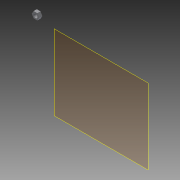
# Autodesk Inventor part: m5_nut
Saved by Autodesk Inventor 2014 (Build 180170000, 170)
## iProperties
Created: 2014-02-14
Part Number: m5_nut
Material: Generic
Document SubType Name: Modeling
Designer: stephen
Density: 1 g/cm^3
Appearance: Default
Author: stephen
Autodesk Inventor part; units mm, degrees
ref_plane "YZ Plane" through (0, 0, 0) normal (1, 0, 0) x (0, 1, 0)
ref_plane "XZ Plane" through (0, 0, 0) normal (0, 1, 0) x (-1, 0, 0)
ref_plane "XY Plane" through (0, 0, 0) normal (0, 0, 1) x (1, 0, 0)
ref_plane "Work Plane2" through (-37.9568, -6.3739, 16.6205) normal (0.2239, -0.0206, 0.9744) x (0.9746, 0.0023, -0.2239)
sketch "Sketch1" plane through (-37.9568, -6.3739, 16.6205) normal (0.2239, -0.0206, 0.9744) x (0.9746, 0.0023, -0.2239)
  circle A0 centre (40.7292, 6.1193) radius 2.5
  line L0 (45.348, 6.1193) -> (43.0386, 2.1193)
  line L1 (43.0386, 2.1193) -> (38.4198, 2.1193)
  line L2 (38.4198, 2.1193) -> (36.1104, 6.1193)
  line L3 (36.1104, 6.1193) -> (38.4198, 10.1193)
  line L4 (38.4198, 10.1193) -> (43.0386, 10.1193)
  line L5 (43.0386, 10.1193) -> (45.348, 6.1193)
  point P0 (40.7292, 6.1193)
  dimension "d0" = 5
  dimension "d1" = 8
  constraints: 12 end point, 2 coincident, 1 centre point, 13 other
  measures "d0" diameter of A0
  measures "d1" distance between parallel lines of L1 L4
extrude "Extrusion1" add sketch "Sketch1" along normal blind 4
body "Solid1"
